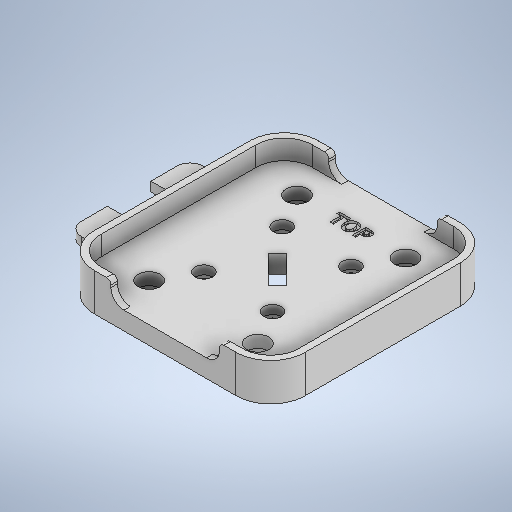
# Autodesk Inventor part: Pin-Cradle
Saved by Autodesk Inventor 2025 (Build 290162000, 162)
## iProperties
Created: 2025-03-04
Part Number: Pin-Cradle
Material: Generic
Document SubType Name: Modeling
Designer: maxsm
Density: 1 g/cm^3
Appearance: Default
Author: maxsm
Autodesk Inventor part; units mm, degrees
ref_plane "YZ Plane" through (0, 0, 0) normal (1, 0, 0) x (0, 1, 0)
ref_plane "XZ Plane" through (0, 0, 0) normal (0, 1, 0) x (-1, 0, 0)
ref_plane "XY Plane" through (0, 0, 0) normal (0, 0, 1) x (1, 0, 0)
sketch "Sketch1" plane through (0, 0, 0) normal (0, 1, 0) x (-1, 0, 0)
  line L0 (16.25, 25.8) -> (-16.25, 25.8)
  line L1 (-24.25, 17.8) -> (-24.25, -17.8)
  line L2 (-16.25, -25.8) -> (16.25, -25.8)
  line L3 (24.25, -17.8) -> (24.25, 17.8)
  line L4 (24.25, 25.8) -> (-24.25, -25.8) construction
  line L5 (-24.25, 25.8) -> (24.25, -25.8) construction
  arc A0 (24.25, 17.8) -> (16.25, 25.8) centre (16.25, 17.8) ccw
  arc A1 (16.25, -25.8) -> (24.25, -17.8) centre (16.25, -17.8) ccw
  arc A2 (-24.25, -17.8) -> (-16.25, -25.8) centre (-16.25, -17.8) ccw
  arc A3 (-16.25, 25.8) -> (-24.25, 17.8) centre (-16.25, 17.8) ccw
  point P0 (0, 0)
  dimension "d1" = 48.5
  dimension "d2" = 51.6
  dimension "d3" = 8
  constraints: 12 end point, 8 point on circle, 8 point on line, 8 tangent, 4 centre point, 3 equal radius, 2 midpoint, 2 parallel, 1 horizontal, 1 perpendicular
  measures "d1" distance between parallel lines of L1 L3
  measures "d2" distance between parallel lines of L0 L2
  measures "d3" radius of A0
extrude "Extrusion1" add sketch "Sketch1" along normal blind 6
shell "Shell1" thickness 1.5 removed faces 1 at (8.0833, 6, -5.9333)
thicken "Thicken1" operation add thickness 2.65 both sides no extend neighbours no toward (0, -1, 0) faces at (8.0833, 0, -5.9333)
sketch "Sketch2" plane through (-16.25, 1.5, -24.3) normal (0, 1, 0) x (1, 0, 0)
  line L0 (18.3713, -28.5426) -> (12.0074, -22.1787)
  line L1 (12.0074, -22.1787) -> (14.1287, -20.0574)
  line L2 (14.1287, -20.0574) -> (20.4926, -26.4213)
  line L3 (20.4926, -26.4213) -> (18.3713, -28.5426)
  line L4 (18.3713, -28.5426) -> (14.1287, -20.0574) construction
  line L5 (12.0074, -22.1787) -> (20.4926, -26.4213) construction
  line L6 (18.3713, -28.5426) -> (27.3713, -28.5426) construction
  line L7 (-6.5, -42.1) -> (-6.5, -6.5) construction
  line L8 (0, 0) -> (32.5, 0) construction
  circle A0 centre (8.35, -15.3) radius 1.05
  circle A1 centre (8.35, -33.3) radius 1.05
  line L9 (-17.7, -24.3) -> (50.2, -24.3) projected
  circle A2 centre (24.15, -15.3) radius 1.05
  circle A3 centre (24.15, -33.3) radius 1.05
  line L10 (16.25, 11.82) -> (16.25, -60.42) projected
  point P0 (16.25, -24.3)
  point P1 (16.25, -24.3)
  point P2 (16.25, -24.3)
  dimension "d12" = 9
  dimension "d13" = 135
  dimension "d14" = 3
  dimension "d15" = 22.75
  dimension "d16" = 24.3
  dimension "d19" = 7.9
  dimension "d20" = 2.1
  dimension "d21" = 18
  constraints: 14 end point, 4 centre point, 4 midpoint, 3 equal radius, 2 parallel, 2 symmetric about line, 2 vertical alignment, 1 equal length, 1 horizontal, 1 horizontal alignment, 1 perpendicular
  measures "d12" distance of L0.start L0.end
  measures "d13" angle of L6 L0
  measures "d14" distance of L0.end L1.end
  measures "d15" distance from line of point (16.25, -24.3) L7
  measures "d16" distance from line of point (16.25, -24.3) L8
  measures "d19" horizontal distance of point (16.25, -24.3) A0.centre
  measures "d20" diameter of A0
  measures "d21" distance of A1.centre A0.centre
extrude "Extrusion2" cut sketch "Sketch2" against normal through all
sketch "Sketch3" plane through (-16.25, 1.5, -24.3) normal (0, 1, 0) x (1, 0, 0)
  circle A0 centre (3.75, -7.3) radius 2.5
  circle A1 centre (28.75, -7.3) radius 2.5
  circle A2 centre (3.75, -41.3) radius 2.5
  circle A3 centre (28.75, -41.3) radius 2.5
  point P0 (16.25, -24.3)
  dimension "d22" = 5
  dimension "d23" = 25
  dimension "d24" = 34
  dimension "d25" = 17
  dimension "d26" = 12.5
  constraints: 4 centre point, 3 equal radius, 2 horizontal alignment, 2 vertical alignment
  measures "d22" diameter of A0
  measures "d23" distance of A1.centre A0.centre
  measures "d24" distance of A2.centre A0.centre
  measures "d25" vertical distance of A0.centre point (16.25, -24.3)
  measures "d26" horizontal distance of point (16.25, -24.3) A0.centre
extrude "Extrusion3" cut sketch "Sketch3" against normal blind 2.8
sketch "Sketch4" plane through (-16.25, 1.5, -24.3) normal (0, 1, 0) x (1, 0, 0)
  circle A0 centre (8.35, -15.3) radius 2
  circle A1 centre (8.35, -33.3) radius 1.05 projected
  circle A2 centre (8.35, -33.3) radius 2
  circle A3 centre (8.35, -15.3) radius 1.05 projected
  circle A4 centre (24.15, -15.3) radius 2
  circle A5 centre (24.15, -33.3) radius 2
  circle A6 centre (24.15, -15.3) radius 1.05 projected
  circle A7 centre (24.15, -33.3) radius 1.05 projected
  point P0 (16.25, -24.3)
  dimension "d29" = 4
  constraints: 4 centre point, 3 concentric, 3 equal radius, 1 coincident
  measures "d29" diameter of A0
extrude "Extrusion4" cut sketch "Sketch4" against normal blind 2
sketch "Sketch5" plane through (-16.25, -2.65, 25.8) normal (0, -1, 0) x (1, 0, 0)
  line L0 (-8, -43.6) -> (-8, -8) projected
  line L1 (-8, -39.8) -> (-17.85, -39.8)
  line L2 (-17.85, -39.8) -> (-17.85, -11.8)
  line L3 (-17.85, -11.8) -> (-8, -11.8)
  line L4 (-8, -11.8) -> (-8, -39.8)
  line L5 (-29.52, -25.8) -> (52.17, -25.8) projected
  line L6 (-17.85, -39.8) -> (-8, -39.8)
  line L7 (-8, -39.8) -> (-8, -30.8)
  line L8 (-8, -30.8) -> (-17.85, -30.8)
  line L9 (-17.85, -30.8) -> (-17.85, -39.8)
  circle A0 centre (-10.65, -34.8) radius 1.05
  point P0 (16.25, -25.8)
  point P1 (-8, -11.8)
  point P2 (-8, -30.8)
  point P3 (-17.85, -30.8)
  dimension "d34" = 9.85
  dimension "d35" = 28
  dimension "d37" = 9
  dimension "d38" = 5
  dimension "d40" = 2.1
  dimension "d42" = 2.65
  constraints: 16 end point, 4 parallel, 2 horizontal, 2 perpendicular, 2 point on line, 1 centre point, 1 other
  measures "d34" distance between parallel lines of L0 L2
  measures "d35" distance between parallel lines of L3 L1
  measures "d37" distance between parallel lines of L1 L8
  measures "d38" distance from line of A0.centre L1
  measures "d40" diameter of A0
  measures "d42" distance from line of L0 A0.centre
extrude "Extrusion5" add sketch "Sketch5" against normal blind 2.15 contours L1 L2 L8 L0
fillet "Fillet1" radius 3 1 edges at (-34.1, -1.575, -14)
mirror "Mirror1" about plane through (0, 0, 0) normal (0, 0, 1) of "Extrusion5", "Fillet1"
sketch "Sketch6" plane through (-16.25, 6, 25.8) normal (0, 0, 1) x (1, 0, 0)
  line L0 (32.5, 0) -> (0, 0) projected
  line L1 (3.75, 0) -> (28.75, 0)
  line L2 (28.75, 0) -> (28.75, -1.5)
  line L3 (25.75, -4.5) -> (6.75, -4.5)
  line L4 (3.75, -1.5) -> (3.75, 0)
  line L5 (16.25, -4.5) -> (16.25, 4.7143) construction
  line L6 (32.5, -8.65) -> (0, -8.65) projected
  line L7 (0, -8.65) -> (0, 0) projected
  line L8 (0, 0) -> (32.5, 0) projected
  line L9 (32.5, 0) -> (32.5, -8.65) projected
  arc A0 (3.75, -1.5) -> (6.75, -4.5) centre (6.75, -1.5) ccw
  arc A1 (25.75, -4.5) -> (28.75, -1.5) centre (25.75, -1.5) ccw
  point P0 (16.25, -6)
  dimension "d43" = 25
  dimension "d44" = 4.5
  dimension "d45" = 3
  constraints: 10 end point, 4 point on circle, 4 tangent, 2 centre point, 2 parallel, 1 equal radius, 1 horizontal, 1 midpoint, 1 perpendicular, 1 point on line, 1 vertical, 1 vertical alignment
  measures "d43" distance between parallel lines of L2 L4
  measures "d44" distance between parallel lines of L3 L0
  measures "d45" radius of A0
extrude "Extrusion6" cut sketch "Sketch6" against normal through all contours L2 A1 L3 A0 L4 L0
fillet "Fillet2" radius 1 4 edges at (-12.5, 6, 25.05) (12.5, 6, 25.05) (-12.5, 6, -25.05) (12.5, 6, -25.05)
sketch "Sketch7" plane through (22.75, 1.5, 17.8) normal (0, 1, 0) x (1, 0, 0)
  line L0 (-27.75, 36.8) -> (-17.75, 36.8) construction
  line L1 (-17.75, 36.8) -> (-17.75, 32.8) construction
  line L2 (-17.75, 32.8) -> (-27.75, 32.8) construction
  line L3 (-27.75, 32.8) -> (-27.75, 36.8) construction
  line L4 (-22.75, 36.8) -> (-22.75, 32.8) construction
  line L5 (-27.75, 34.8) -> (-17.75, 34.8) construction
  circle A0 centre (-35.25, 34.8) radius 2.5 projected
  line L6 (-26.125, 33.275) -> (-26.125, 35.7442)
  line L7 (-26.125, 35.7442) -> (-27.0272, 35.7442)
  line L8 (-27.0272, 35.7442) -> (-27.0272, 36.325)
  line L9 (-27.0272, 36.325) -> (-24.4567, 36.325)
  line L10 (-24.4567, 36.325) -> (-24.4567, 35.7442)
  line L11 (-24.4567, 35.7442) -> (-25.3588, 35.7442)
  line L12 (-25.3588, 35.7442) -> (-25.3588, 33.275)
  line L13 (-25.3588, 33.275) -> (-26.125, 33.275)
  spline S0 degree 2 poles (-21.3671, 34.8) (-21.3671, 34.0585) (-22.158, 33.2107) (-22.8452, 33.2107) knots 0 0 0 1 2 2 2
  spline S1 degree 2 poles (-22.8452, 33.2107) (-23.5347, 33.2107) (-24.3207, 34.0684) (-24.3207, 34.8) knots 0 0 0 1 2 2 2
  spline S2 degree 2 poles (-24.3207, 34.8) (-24.3207, 35.5341) (-23.5347, 36.3893) (-22.8452, 36.3893) knots 0 0 0 1 2 2 2
  spline S3 degree 2 poles (-22.8452, 36.3893) (-22.158, 36.3893) (-21.3671, 35.539) (-21.3671, 34.8) knots 0 0 0 1 2 2 2
  spline S4 degree 2 poles (-22.158, 34.8) (-22.158, 35.0744) (-22.2693, 35.4575) (-22.3657, 35.5786) knots 0 0 0 1 2 2 2
  spline S5 degree 2 poles (-22.3657, 35.5786) (-22.4621, 35.7046) (-22.7092, 35.8134) (-22.8427, 35.8134) knots 0 0 0 1 2 2 2
  spline S6 degree 2 poles (-22.8427, 35.8134) (-22.9836, 35.8134) (-23.2134, 35.712) (-23.3197, 35.5835) knots 0 0 0 1 2 2 2
  spline S7 degree 2 poles (-23.3197, 35.5835) (-23.4136, 35.4649) (-23.5298, 35.0719) (-23.5298, 34.8) knots 0 0 0 1 2 2 2
  spline S8 degree 2 poles (-23.5298, 34.8) (-23.5298, 34.5182) (-23.4186, 34.1475) (-23.3222, 34.0214) knots 0 0 0 1 2 2 2
  spline S9 degree 2 poles (-23.3222, 34.0214) (-23.2258, 33.8954) (-22.9762, 33.7866) (-22.8427, 33.7866) knots 0 0 0 1 2 2 2
  spline S10 degree 2 poles (-22.8427, 33.7866) (-22.7067, 33.7866) (-22.4546, 33.9028) (-22.3632, 34.0264) knots 0 0 0 1 2 2 2
  spline S11 degree 2 poles (-22.3632, 34.0264) (-22.2643, 34.1598) (-22.158, 34.5133) (-22.158, 34.8) knots 0 0 0 1 2 2 2
  spline S12 degree 2 poles (-18.5668, 35.3635) (-18.5668, 35.151) (-18.7027, 34.7654) (-18.8287, 34.6369) knots 0 0 0 1 2 2 2
  spline S13 degree 2 poles (-18.8287, 34.6369) (-18.9054, 34.5553) (-19.0932, 34.4218) (-19.2044, 34.3749) knots 0 0 0 1 2 2 2
  spline S14 degree 2 poles (-19.2044, 34.3749) (-19.3181, 34.3279) (-19.5826, 34.2735) (-19.7457, 34.2735) knots 0 0 0 1 2 2 2
  line L14 (-19.7457, 34.2735) -> (-20.1461, 34.2735)
  line L15 (-20.1461, 34.2735) -> (-20.1461, 33.275)
  line L16 (-20.1461, 33.275) -> (-20.9123, 33.275)
  line L17 (-20.9123, 33.275) -> (-20.9123, 36.325)
  line L18 (-20.9123, 36.325) -> (-19.7284, 36.325)
  spline S15 degree 2 poles (-19.7284, 36.325) (-19.4664, 36.325) (-19.0833, 36.2286) (-18.9276, 36.1248) knots 0 0 0 1 2 2 2
  spline S16 degree 2 poles (-18.9276, 36.1248) (-18.7546, 36.0086) (-18.5668, 35.628) (-18.5668, 35.3635) knots 0 0 0 1 2 2 2
  spline S17 degree 2 poles (-19.3527, 35.3438) (-19.3527, 35.4748) (-19.4763, 35.6601) (-19.5604, 35.6947) knots 0 0 0 1 2 2 2
  spline S18 degree 2 poles (-19.5604, 35.6947) (-19.6691, 35.7417) (-19.8668, 35.7565) (-20.0374, 35.7565) knots 0 0 0 1 2 2 2
  line L19 (-20.0374, 35.7565) -> (-20.1461, 35.7565)
  line L20 (-20.1461, 35.7565) -> (-20.1461, 34.842)
  line L21 (-20.1461, 34.842) -> (-20.0918, 34.842)
  spline S19 degree 2 poles (-20.0918, 34.842) (-19.9855, 34.842) (-19.7927, 34.847) (-19.721, 34.8593) knots 0 0 0 1 2 2 2
  spline S20 degree 2 poles (-19.721, 34.8593) (-19.6592, 34.8692) (-19.5233, 34.9285) (-19.4862, 34.9656) knots 0 0 0 1 2 2 2
  spline S21 degree 2 poles (-19.4862, 34.9656) (-19.4071, 35.0397) (-19.3527, 35.2053) (-19.3527, 35.3438) knots 0 0 0 1 2 2 2
  point P0 (-22.75, 17.8)
  point P1 (-22.75, 34.8)
  dimension "d49" = 10
  dimension "d50" = 4
  constraints: 5 midpoint, 4 end point, 1 horizontal alignment, 1 perpendicular, 1 vertical, 1 vertical alignment, 3 other
  measures "d49" distance between parallel lines of L1 L3
  measures "d50" distance between parallel lines of L2 L0
extrude "Extrusion7" cut sketch "Sketch7" against normal blind 0.5 contours L6 L7 L8 L9 L10 L11 L12 L13 | S0 S1 S2 S3 | S12 S13 S14 L14 L15 L16 L17 L18 S15 S16
equation "\"d25\" = 0.5 * d24"
equation "\"d26\" = 0.5 * d23"
body "Solid1"
